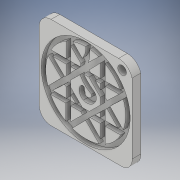
# Autodesk Inventor part: fma key chain
Saved by Autodesk Inventor 2017 (Build 210142000, 142)
## iProperties
Created: 2017-10-02
Part Number: fma key chain
Material: Generic
Document SubType Name: Modeling
Designer: Hamza
Density: 1 g/cm^3
Appearance: Default
Author: Hamza
Autodesk Inventor part; units mm, degrees
ref_plane "YZ Plane" through (0, 0, 0) normal (1, 0, 0) x (0, 1, 0)
ref_plane "XZ Plane" through (0, 0, 0) normal (0, 1, 0) x (-1, 0, 0)
ref_plane "XY Plane" through (0, 0, 0) normal (0, 0, 1) x (1, 0, 0)
sketch "Sketch1" plane through (0, 0, 0) normal (0, 0, 1) x (1, 0, 0)
  line L0 (0, 0) -> (76.2, 0)
  line L1 (76.2, 0) -> (76.2, 76.2)
  line L2 (76.2, 76.2) -> (0, 76.2)
  line L3 (0, 76.2) -> (0, 0)
  line L4 (2.2528, 73.2748) -> (74.5621, 73.2748) construction
  line L5 (74.5621, 73.2748) -> (74.5621, 0.9654) construction
  line L6 (74.5621, 0.9654) -> (2.2528, 0.9654) construction
  line L7 (2.2528, 0.9654) -> (2.2528, 73.2748) construction
  dimension "d0" = 76.2
  dimension "d1" = 76.2
  constraints: 8 end point, 2 parallel, 1 horizontal, 1 perpendicular, 2 other
  measures "d0" distance of L2.end L1.end
  measures "d1" distance of L1.end L0.end
extrude "Extrusion1" add sketch "Sketch1" along normal blind 6.35
sketch "Sketch4" plane through (0, 0, 6.35) normal (0, 0, 1) x (1, 0, 0)
  circle A0 centre (37.9936, 35.4133) radius 32.6267
  arc A1 (39.8332, 55.5329) -> (41.0153, 64.5774) centre (21.7277, 62.4987) ccw
  line L0 (39.8332, 55.5329) -> (47.7065, 63.078)
  line L1 (35.4215, 56.0068) -> (28.5545, 63.1726)
  line L2 (27.0645, 59.661) -> (27.0645, 49.8358)
  line L3 (27.0645, 49.8358) -> (33.9998, 49.8358)
  line L4 (33.9998, 49.8358) -> (34.4926, 52.1967)
  line L5 (34.4926, 52.1967) -> (27.0645, 59.661)
  line L6 (48.8306, 59.661) -> (48.8306, 49.8358)
  line L7 (48.8306, 49.8358) -> (41.7025, 49.8358)
  line L8 (41.7025, 49.8358) -> (40.4884, 51.0559)
  line L9 (40.4884, 51.0559) -> (48.8306, 59.661)
  line L10 (52.2851, 61.0147) -> (52.2851, 49.8698)
  line L11 (52.2851, 49.8698) -> (63.5022, 49.8698)
  line L12 (52.2851, 46.6403) -> (62.508, 46.6403)
  line L13 (62.508, 46.6403) -> (53.7962, 38.3039)
  line L14 (53.7962, 38.3039) -> (52.2851, 39.3338)
  line L15 (52.2851, 39.3338) -> (52.2851, 46.6403)
  line L16 (65.6602, 45.121) -> (55.7896, 35.6757)
  line L17 (55.7896, 35.6757) -> (65.5707, 25.4541)
  line L18 (52.2851, 31.7758) -> (53.6941, 33.1242)
  line L19 (53.6941, 33.1242) -> (61.6989, 24.759)
  line L20 (61.6989, 24.759) -> (52.2851, 24.759)
  line L21 (52.2851, 24.759) -> (52.2851, 31.7758)
  line L22 (48.6187, 28.2674) -> (48.6187, 24.759)
  line L23 (48.6187, 24.759) -> (44.9523, 24.759)
  line L24 (48.6187, 28.2674) -> (44.9523, 24.759)
  line L25 (63.6819, 21.2785) -> (52.2851, 21.2785)
  line L26 (52.2851, 21.2785) -> (52.2851, 9.8118)
  line L27 (41.3151, 21.2785) -> (40.3692, 20.3734)
  line L28 (40.3692, 20.3734) -> (48.8306, 11.531)
  line L29 (48.8306, 11.531) -> (48.8306, 21.2785)
  line L30 (48.8306, 21.2785) -> (41.3151, 21.2785)
  line L31 (28.1116, 7.8085) -> (37.9638, 17.8289)
  line L32 (37.9638, 17.8289) -> (47.8757, 7.8085)
  line L33 (45.0728, 46.6403) -> (48.8306, 46.6403)
  line L34 (48.8306, 46.6403) -> (48.8306, 42.4948)
  line L35 (48.8306, 42.4948) -> (45.0728, 46.6403)
  line L36 (27.0645, 21.5303) -> (27.0645, 11.531)
  line L37 (27.0645, 11.531) -> (35.6907, 20.0638)
  line L38 (35.6907, 20.0638) -> (34.3025, 21.5303)
  line L39 (34.3025, 21.5303) -> (27.0645, 21.5303)
  line L40 (27.0645, 24.759) -> (27.0645, 28.5453)
  line L41 (27.0645, 28.5453) -> (31.2461, 24.759)
  line L42 (31.2461, 24.759) -> (27.0645, 24.759)
  line L43 (23.5078, 9.9213) -> (23.5078, 21.5303)
  line L44 (23.5078, 21.5303) -> (12.1684, 21.5303)
  line L45 (22.338, 32.8248) -> (13.8176, 24.759)
  line L46 (13.8176, 24.759) -> (23.8582, 24.759)
  line L47 (23.8582, 24.759) -> (23.8582, 32.0259)
  line L48 (23.8582, 32.0259) -> (22.338, 32.8248)
  line L49 (10.2893, 25.8139) -> (20.1341, 35.7908)
  line L50 (20.1341, 35.7908) -> (10.3737, 45.2529)
  line L51 (13.7843, 46.4428) -> (23.8582, 46.4428)
  line L52 (23.8582, 46.4428) -> (23.8582, 39.1403)
  line L53 (23.8582, 39.1403) -> (22.6271, 37.8703)
  line L54 (22.6271, 37.8703) -> (13.7843, 46.4428)
  line L55 (12.4851, 49.8698) -> (23.8582, 49.8698)
  line L56 (23.8582, 49.8698) -> (23.8582, 61.1012)
  line L57 (36.527, 46.4405) -> (40.3463, 46.4405)
  line L58 (40.3463, 46.4405) -> (48.8077, 37.868)
  line L59 (48.8077, 37.868) -> (48.8077, 32.9029)
  line L60 (48.8077, 32.9029) -> (40.5546, 24.7568)
  line L61 (40.5546, 24.7568) -> (35.5243, 24.7568)
  line L62 (35.5243, 24.7568) -> (27.0415, 33.3082)
  line L63 (27.0415, 33.3082) -> (27.0415, 37.9669)
  line L64 (27.0415, 37.9669) -> (33.8336, 44.7045)
  arc A2 (37.3088, 37.4861) -> (34.5624, 38.4061) centre (35.7291, 37.3295) ccw
  arc A3 (35.4215, 56.0068) -> (38.0897, 64.7334) centre (24.8347, 64.015) ccw
  line L65 (30.7856, 46.4428) -> (27.0645, 46.4428)
  line L66 (27.0645, 46.4428) -> (27.0645, 42.7915)
  line L67 (27.0645, 42.7915) -> (30.7856, 46.4428)
  arc A4 (38.0897, 64.7334) -> (28.5545, 63.1726) centre (37.9936, 35.4133) ccw
  arc A5 (23.8582, 61.1012) -> (12.4851, 49.8698) centre (37.9936, 35.4133) ccw
  arc A6 (10.3737, 45.2529) -> (10.2893, 25.8139) centre (37.9936, 35.4133) ccw
  arc A7 (12.1684, 21.5303) -> (23.5078, 9.9213) centre (37.9936, 35.4133) ccw
  arc A8 (28.1116, 7.8085) -> (47.8757, 7.8085) centre (37.9936, 35.4133) ccw
  arc A9 (52.2851, 9.8118) -> (63.6819, 21.2785) centre (37.9936, 35.4133) ccw
  arc A10 (65.5707, 25.4541) -> (65.6602, 45.121) centre (37.9936, 35.4133) ccw
  arc A11 (63.5022, 49.8698) -> (52.2851, 61.0147) centre (37.9936, 35.4133) ccw
  arc A12 (47.7065, 63.078) -> (41.0153, 64.5774) centre (37.9936, 35.4133) ccw
  arc A13 (33.8336, 44.7045) -> (42.2384, 36.5279) centre (50.4148, 53.3406) ccw
  arc A14 (36.527, 46.4405) -> (44.3063, 39.1864) centre (64.5241, 68.6662) ccw
  arc A15 (41.9514, 34.4186) -> (42.2384, 36.5279) centre (40.1326, 35.7402) ccw
  arc A16 (37.6546, 33.9983) -> (41.9514, 34.4186) centre (39.6248, 36.0309) ccw
  line L68 (37.6546, 33.9983) -> (37.3088, 37.4861)
  arc A17 (44.5995, 32.3578) -> (44.3063, 39.1864) centre (40.7913, 35.6149) ccw
  arc A18 (36.3329, 29.7841) -> (44.5995, 32.3578) centre (38.9394, 35.9748) ccw
  arc A19 (34.5624, 38.4061) -> (36.3329, 29.7841) centre (38.5448, 34.731) ccw
  arc A20 (37.1687, 38.8991) -> (37.0823, 38.9844) centre (36.1383, 37.9413) ccw
  point P0 (0, 0)
  dimension "d39" = 3.2295
  dimension "d40" = 3.4545
  dimension "d41" = 3.4545
  dimension "d42" = 3.175
  dimension "d43" = 3.2062
  dimension "d44" = 3.393
  dimension "d45" = 3.427
  dimension "d46" = 3.2062
  dimension "d47" = 3.2062
  dimension "d48" = 3.5566
  dimension "d49" = 3.2287
  dimension "d50" = 3.4545
  dimension "d51" = 3.4805
  dimension "d52" = 3.6664
  constraints: 138 end point, 41 point on circle, 28 perpendicular, 27 point on line, 21 centre point, 7 parallel, 6 horizontal, 3 tangent, 3 vertical, 1 coincident
  measures "d39" distance between parallel lines of L12 L11
  measures "d40" distance between parallel lines of L34 L15
  measures "d41" distance between parallel lines of L10 L6
  measures "d42" diameter of A2
  measures "d43" distance between parallel lines of L56 L2
  measures "d44" distance between parallel lines of L65 L3
  measures "d45" distance between parallel lines of L51 L55
  measures "d46" distance between parallel lines of L66 L52
  measures "d47" distance between parallel lines of L47 L40
  measures "d48" distance between parallel lines of L43 L36
  measures "d49" distance between parallel lines of L42 L39
  measures "d50" distance between parallel lines of L26 L29
  measures "d51" distance between parallel lines of L30 L23
  measures "d52" distance between parallel lines of L21 L22
extrude "Extrusion2" cut sketch "Sketch4" against normal blind 3.175
sketch "Sketch5" plane through (0, 0, 6.35) normal (0, 0, 1) x (1, 0, 0)
  line L0 (3.9067, 61.5796) -> (3.9067, 10.1455)
  line L1 (12.4086, 1.7144) -> (63.8436, 1.7144)
  arc A0 (3.9067, 10.1455) -> (12.4086, 1.7144) centre (12.4086, 10.2166) ccw
  line L2 (72.0119, 61.6228) -> (72.0119, 10.1887)
  arc A1 (63.8436, 1.7144) -> (72.0119, 10.1887) centre (64.2266, 9.519) ccw
  line L3 (12.5886, 69.2455) -> (62.1529, 69.2455)
  arc A2 (12.5886, 69.2455) -> (3.9067, 61.5796) centre (12.5886, 60.4963) ccw
  arc A3 (72.0119, 61.6228) -> (62.1529, 69.2455) centre (62.1529, 59.0584) ccw
  circle A4 centre (64.7183, 63.0004) radius 3.175
  point P0 (0, 0)
  dimension "d55" = 51.4341
  dimension "d56" = 51.435
  dimension "d57" = 6.35
  constraints: 8 end point, 8 point on circle, 5 centre point, 3 tangent, 2 horizontal, 2 vertical
  measures "d55" distance of L0.start L0.end
  measures "d56" distance of L1.start L1.end
  measures "d57" diameter of A4
extrude "Extrusion3" cut sketch "Sketch5" against normal through all contours A4
extrude "Extrusion4" cut sketch "Sketch5" against normal through all keep common part
body "Solid1"
